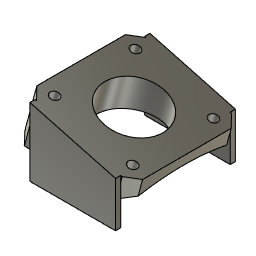
motor mount (Autodesk Fusion 360 design; units mm, degrees)
Autodesk Fusion 360 part; units mm, degrees
sketch "Sketch5" plane through (0, 0, 0) normal (1, 0, 0) x (0, 1, 0)
  line L0 (-20, 0) -> (20, 0)
  arc A0 (20, 0) -> (-20, 0) centre (0, -65.1667) ccw
  line L1 (-9.145, 3) -> (16.9339, 3) construction
  line L2 (-20, 0) -> (20, 0)
  line L3 (20, 0) -> (20, -3)
  line L4 (20, -3) -> (-20, -3)
  line L5 (-20, -3) -> (-20, 0)
  dimension "d18" = 3
  dimension "d19" = 40
  dimension "d20" = 3
  constraint horizontal L0
  constraint horizontal L1
  constraint tangent A0 L1
  constraint midpoint origin L0
  constraint horizontal L2
  constraint vertical L3
  constraint horizontal L4
  constraint vertical L5
  measures "d18" distance of L0 L1
  measures "d19" distance of L0.start L0.end
  measures "d20" distance of L0.end L3.end
extrude "Extrude5" add sketch "Sketch5" along normal blind 70 makes body 1
sketch "Sketch6" plane through (0, 0, -3) normal (0, 0, -1) x (1, 0, 0)
  line L0 (0, 20) -> (0, -20)
  line L1 (0, -20) -> (70, -20)
  line L2 (70, -20) -> (70, 20)
  line L3 (70, 20) -> (0, 20)
  line L4 (32.5, -5) -> (47.5, -5)
  arc A0 (47.5, -5) -> (47.5, 5) centre (47.5, 0) ccw
  line L5 (47.5, 5) -> (32.5, 5)
  arc A1 (32.5, 5) -> (32.5, -5) centre (32.5, 0) ccw
  line L6 (32.5, 0) -> (47.5, 0) construction
  line L7 (0, 0) -> (70, 0) construction
  line L8 (40, 5) -> (40, -5) construction
  dimension "d23" = 10
  dimension "d24" = 15
  dimension "d25" = 40
  constraint tangent L4 A0
  constraint tangent A0 L5
  constraint parallel L4 L5
  constraint tangent L5 A1
  constraint tangent L4 A1
  constraint horizontal L6
  constraint coincident L7.start origin
  constraint midpoint L2 L7.end
  constraint collinear L6 L7
  constraint midpoint L5 L8.start
  constraint midpoint L4 L8.end
  measures "d23" distance of L4 L5
  measures "d24" distance of A0.end L5.end
  measures "d25" distance of L0 L8
extrude "Extrude6" cut sketch "Sketch6" against normal through all contours L4 A0 L5 A1 bodies 1
ref_plane "WorkPlane3" through (0, 12.125, 0) normal (-0.965926, 0, 0.258819) x (0, 1, 0)
sketch "Sketch7" plane through (0, 12.125, 0) normal (-0.965926, 0, 0.258819) x (0, 1, 0)
  line L0 (10.375, 0) -> (-34.625, 0)
  line L1 (-34.625, 0) -> (-34.625, -25)
  line L2 (-34.625, -25) -> (10.375, -25)
  line L3 (10.375, -25) -> (10.375, 0)
  line L4 (-10.375, 0) -> (10.375, 0)
  point P0 (-12.125, 0)
  dimension "d28" = 45
  dimension "d29" = 25
  constraint horizontal L0
  constraint vertical L1
  constraint horizontal L2
  constraint vertical L3
  constraint midpoint L0 P0
  measures "d28" distance of L1.end L2.end
  measures "d29" distance of L0.end L1.end
extrude "Extrude7" add sketch "Sketch7" along normal blind 45 bodies 1
extrude "Extrude8" add 1 faces at (-28.9778, -6.6667, 7.7646) along direction (-0.258819, 0, -0.965926) blind 55 on bodies 1 bodies 1
ref_plane "WorkPlane4" through (16.4027, 0, 3) normal (0, 0, 1) x (0, 1, 0)
sketch "Sketch8" plane through (16.4027, 0, 3) normal (0, 0, 1) x (1, 0, 0)
  line L0 (16.0973, 5) -> (31.0973, 5)
  spline S0 degree 3 poles (31.0973, 5) (31.7254, 5) (32.3951, 4.8744) (33.627, 4.3641) (34.189, 3.9793) (35.0767, 3.0917) (35.4614, 2.5296) (35.9718, 1.2978) (36.0973, 0.6281) (36.0973, -0.6281) (35.9718, -1.2978) (35.4614, -2.5296) (35.0767, -3.0917) (34.189, -3.9793) (33.627, -4.3641) (32.3951, -4.8744) (31.7254, -5) (31.0973, -5) knots -1.507328 -1.507328 -1.507328 -1.507328 -1.318912 -1.318912 -1.130496 -1.130496 -0.94208 -0.94208 -0.753664 -0.753664 -0.565248 -0.565248 -0.376832 -0.376832 -0.188416 -0.188416 0 0 0 0
  line L1 (31.0973, -5) -> (16.0973, -5)
  spline S1 degree 3 poles (16.0973, -5) (15.4693, -5) (14.7995, -4.8744) (13.5677, -4.3641) (13.0056, -3.9793) (12.118, -3.0917) (11.7332, -2.5296) (11.2229, -1.2978) (11.0973, -0.6281) (11.0973, 0.6281) (11.2229, 1.2978) (11.7332, 2.5296) (12.118, 3.0917) (13.0056, 3.9793) (13.5677, 4.3641) (14.7995, 4.8744) (15.4693, 5) (16.0973, 5) knots 0 0 0 0 0.188416 0.188416 0.376832 0.376832 0.565248 0.565248 0.753664 0.753664 0.94208 0.94208 1.130496 1.130496 1.318912 1.318912 1.507328 1.507328 1.507328 1.507328
  line L2 (23.5973, 5) -> (23.5973, -5) construction
  circle A0 centre (23.5973, 0) radius 16
  circle A1 centre (23.5973, 0) radius 13
  dimension "d35" = 32
  dimension "d36" = 26
  constraint midpoint L0 L2.start
  constraint midpoint L1 L2.end
  constraint midpoint L2 A0.centre
  constraint concentric A0 A1
  measures "d35" diameter of A0
  measures "d36" diameter of A1
ref_plane "WorkPlane5" through (40, 0, 3) normal (0.258819, 0, 0.965926) x (0, -1, 0)
ref_plane "WorkPlane6" through (42.0706, 0, 10.7274) normal (0.258819, 0, 0.965926) x (0, -1, 0)
sketch "Sketch10" plane through (42.0706, 0, 10.7274) normal (0.258819, 0, 0.965926) x (0, -1, 0)
  line L0 (21, -21) -> (-21, 21) construction
  line L1 (21, -21) -> (-21, -21)
  line L2 (-21, -21) -> (-21, 21)
  line L3 (-21, 21) -> (21, 21)
  line L4 (21, 21) -> (21, -21)
  line L5 (21, -17) -> (17, -21)
  line L6 (-17, -21) -> (-21, -17)
  line L7 (-21, 17) -> (-17, 21)
  line L8 (21, 17) -> (17, 21)
  line L9 (-21, -17) -> (-23, -17)
  line L10 (-23, -17) -> (-23, 17)
  line L11 (-23, 17) -> (-21, 17)
  line L12 (-21, 17) -> (-21, -17)
  line L13 (21, -17) -> (23, -17)
  line L14 (23, -17) -> (23, 17)
  line L15 (23, 17) -> (21, 17)
  line L16 (21, 17) -> (21, -17)
  circle A0 centre (0, 0) radius 11.5
  line L17 (15.5, -15.5) -> (-15.5, -15.5) construction
  line L18 (-15.5, -15.5) -> (-15.5, 15.5) construction
  line L19 (-15.5, 15.5) -> (15.5, 15.5) construction
  line L20 (15.5, 15.5) -> (15.5, -15.5) construction
  line L21 (0, -21) -> (0, -15.5) construction
  line L22 (0, 15.5) -> (0, 21) construction
  circle A1 centre (15.5, -15.5) radius 1.75
  circle A2 centre (-15.5, -15.5) radius 1.75
  circle A3 centre (15.5, 15.5) radius 1.75
  circle A4 centre (-15.5, 15.5) radius 1.75
  circle A5 centre (15.5, -15.5) radius 3.25
  circle A6 centre (-15.5, -15.5) radius 3.25
  circle A7 centre (-15.5, 15.5) radius 3.25
  circle A8 centre (15.5, 15.5) radius 3.25
  dimension "d64" = 42
  dimension "d65" = 4
  dimension "d66" = 2
  dimension "d67" = 2
  dimension "d75" = 23
  dimension "d76" = 31
  dimension "d77" = 3.5
  dimension "d78" = 6.5
  constraint midpoint A0.centre L0
  constraint horizontal L1
  constraint vertical L2
  constraint horizontal L3
  constraint vertical L4
  constraint equal L1 L2
  constraint coincident L4 L5.start
  constraint coincident L1 L5.end
  constraint perpendicular L0 L5
  constraint coincident L1 L6.start
  constraint coincident L2 L6.end
  constraint coincident L2 L7.start
  constraint coincident L3 L7.end
  constraint perpendicular L0 L7
  constraint coincident L4 L8.start
  constraint coincident L3 L8.end
  constraint perpendicular L7 L8
  constraint perpendicular L5 L6
  constraint equal L5 L6
  constraint equal L6 L7
  constraint equal L7 L8
  constraint horizontal L9
  constraint vertical L10
  constraint horizontal L11
  constraint vertical L12
  constraint horizontal L13
  constraint vertical L14
  constraint horizontal L15
  constraint vertical L16
  constraint coincident L7.start L11.end
  constraint coincident A0.centre origin
  constraint horizontal L17
  constraint vertical L18
  constraint horizontal L19
  constraint vertical L20
  constraint coincident L0 L18.end
  constraint coincident L0 L17.start
  constraint midpoint L1 L21.start
  constraint midpoint L17 L21.end
  constraint midpoint L19 L22.start
  constraint midpoint L3 L22.end
  constraint equal L21 L22
  constraint coincident L17.start L20.end
  constraint coincident L17.end L18.start
  constraint coincident L19.end L20.start
  constraint coincident L18.end L19.start
  constraint equal A3 A4
  constraint equal A1 A3
  constraint equal A1 A2
  constraint concentric A1 A5
  constraint concentric A2 A6
  constraint equal A5 A8
  constraint equal A5 A6
  constraint equal A6 A7
  measures "d64" distance of L0.end L1.end
  measures "d65" vertical distance of L7.start L7.end
  measures "d66" distance of L8.start L14.end
  measures "d67" distance of L10.end L7.start
  measures "d75" diameter of A0
  measures "d76" distance of L17.end L18.end
  measures "d77" diameter of A2
  measures "d78" diameter of A7
extrude "Extrude16" add sketch "Sketch10" along normal up to surface from surface at 2 separate body contours L1 L2 L3 L4 L5 L6 L7 L8 L12 L16 | A5 | A6 | A7 | A8 end surface at (34.1667, -15.0749, 1.3122) on bodies 1 makes body 2
sketch "Sketch13" plane through (0, 0, -3) normal (0, 0, -1) x (1, 0, 0)
  line L0 (32.5, 5) -> (47.5, 5)
  arc A0 (47.5, -5) -> (47.5, 5) centre (47.5, 0) ccw
  line L1 (47.5, -5) -> (32.5, -5)
  arc A1 (32.5, 5) -> (32.5, -5) centre (32.5, 0) ccw
  line L2 (0, 20) -> (0, -20)
  line L3 (0, -20) -> (70, -20)
  line L4 (70, -20) -> (70, 20)
  line L5 (70, 20) -> (0, 20)
  line L6 (25.6498, 23) -> (58.4913, 23)
  line L7 (25.6498, 21) -> (25.6498, 23)
  line L8 (58.4913, 23) -> (58.4913, 21)
  line L9 (58.4913, -21) -> (25.6498, -21)
  line L10 (58.4913, -23) -> (58.4913, -21)
  line L11 (25.6498, -23) -> (58.4913, -23)
  line L12 (21.7861, -21) -> (62.355, -21)
  line L13 (25.6498, -21) -> (25.6498, -23)
  line L14 (58.4913, 21) -> (25.6498, 21)
extrude "Extrude17" add sketch "Sketch13" along normal up to surface and the other way blind -6 contours L6 L7 L8 L14 | L9 L10 L11 L12 L13 end surface through (42.5882, 0, 12.6593) normal (0.258819, 0, 0.965926) offset 0 bodies 2
extrude "Extrude18" cut sketch "Sketch10" against normal through all from surface at -3 contours A5 | A6 | A7 | A8 bodies 2
hidden bodies 1
